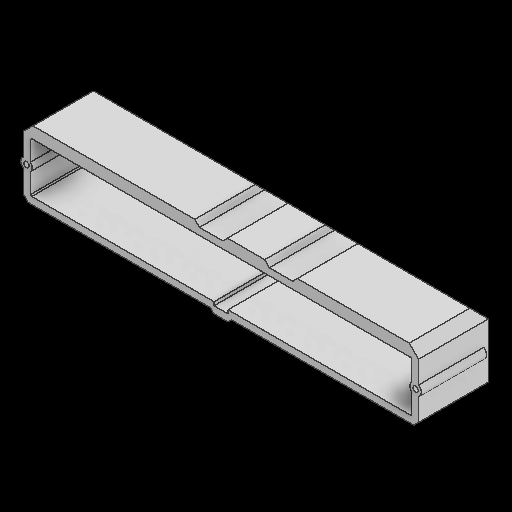
# Autodesk Inventor part: DepthCameraHousing
Saved by Autodesk Inventor 2025.2 (Build 292293000, 293)
## iProperties
Created: 2026-02-04
Part Number: DepthCameraHousing
Material: Generic
Document SubType Name: Modeling
Designer: valer
Density: 1 g/cm^3
Appearance: Default
Author: valer
Autodesk Inventor part; units mm, degrees
ref_plane "YZ Plane" through (0, 0, 0) normal (1, 0, 0) x (0, 1, 0)
ref_plane "XZ Plane" through (0, 0, 0) normal (0, 1, 0) x (-1, 0, 0)
ref_plane "XY Plane" through (0, 0, 0) normal (0, 0, 1) x (1, 0, 0)
sketch "Base" plane through (0, 0, 0) normal (0, 0, 1) x (1, 0, 0)
  line L0 (-81.75, 10.75) -> (81.75, 10.75)
  line L1 (81.75, 10.75) -> (81.75, -10.75)
  line L2 (81.75, -10.75) -> (-81.75, -10.75)
  line L3 (-81.75, -10.75) -> (-81.75, 10.75)
  line L4 (-81.75, 10.75) -> (81.75, -10.75) construction
  line L5 (81.75, 10.75) -> (-81.75, -10.75) construction
  line L6 (-81.75, 10.75) -> (-81.75, 13.75)
  line L7 (-120.4, 0) -> (120.4, 0) construction
  line L8 (0, -19.25) -> (0, 19.25) construction
  line L9 (84.75, 13.75) -> (-84.75, 13.75)
  line L10 (-84.75, 13.75) -> (-84.75, -13.75)
  line L11 (-84.75, -13.75) -> (84.75, -13.75)
  line L12 (84.75, -13.75) -> (84.75, 13.75)
  point P0 (0, 0)
  dimension "d0" = 21.5
  dimension "d1" = 163.5
  dimension "d14" = 3
  constraints: 22 end point, 4 parallel, 2 midpoint, 2 perpendicular, 1 horizontal, 3 other
  measures "d0" distance between parallel lines of L2 L0
  measures "d1" distance of L0.start L0.end
  measures "d14" distance between parallel lines of L0 L9
extrude "BaseFeature" add sketch "Base" along normal blind 27
fillet "InsideFilletsFeature" radius 0.5 4 edges at (-81.75, 10.75, 13.5) (81.75, 10.75, 13.5) (81.75, -10.75, 13.5) (-81.75, -10.75, 13.5)
sketch "Cap" plane through (0, 0, 0) normal (0, 0, -1) x (-1, 0, 0)
  line L0 (84.75, -13.75) -> (-84.75, -13.75) projected
  line L1 (84.75, 13.75) -> (84.75, -13.75) projected
  line L2 (-84.75, 13.75) -> (84.75, 13.75) projected
  line L3 (-84.75, -13.75) -> (-84.75, 13.75) projected
extrude "CapFeature" add sketch "Cap" along normal blind 3
sketch "FrontMount" plane through (0, 0, 0) normal (0, 0, 1) x (1, 0, 0)
  line L0 (-120.4, 0) -> (120.4, 0) construction
  line L1 (0, -19.25) -> (0, 19.25) construction
  circle A0 centre (-83.5, 0) radius 2.5
  circle A1 centre (83.5, 0) radius 2.5
  circle A2 centre (-83.5, 0) radius 1.15
  circle A3 centre (83.5, 0) radius 1.15
  point P0 (0, 0)
  dimension "d11" = 167
  dimension "d12" = 5
  dimension "d13" = 2.3
  constraints: 4 centre point, 2 coincident, 1 equal radius, 1 point on line, 1 symmetric about line, 1 other
  measures "d11" distance of A1.centre A0.centre
  measures "d12" diameter of A0
  measures "d13" diameter of A2
extrude "FrontMountFeature" add sketch "FrontMount" along normal up to surface (27 mm away)
chamfer "SideChamfersFeature" distance 2 angle 45 4 edges at (-84.75, 13.75, 12) (84.75, 13.75, 12) (-84.75, -13.75, 12) (84.75, -13.75, 12)
chamfer "BackChamferFeature" distance 2 angle 45 8 edges at (0, 13.75, -3) (-83.75, 12.75, -3) (-84.75, 0, -3) (-83.75, -12.75, -3) (0, -13.75, -3) (83.75, 12.75, -3) (84.75, 0, -3) (83.75, -12.75, -3)
sketch "FrontMountHoles" plane through (0, 0, 27) normal (0, 0, 1) x (1, 0, 0)
  arc A0 (-84.75, 2.1651) -> (-84.75, -2.1651) centre (-83.5, 0) ccw projected
  arc A1 (84.75, -2.1651) -> (84.75, 2.1651) centre (83.5, 0) ccw projected
  arc A2 (-81.75, -1.7854) -> (-81.75, 1.7854) centre (-83.5, 0) ccw projected
  circle A3 centre (-83.5, 0) radius 1.175
  circle A4 centre (83.5, 0) radius 1.175
  point P0 (0, 0)
  dimension "d20" = 2.35
  dimension "d21" = 2.35
  constraints: 2 centre point, 2 coincident
  measures "d20" diameter of A3
  measures "d21" diameter of A4
extrude "FrontMountHolesFeature" cut sketch "FrontMountHoles" against normal blind 15
sketch "BackEndExtrusion" plane through (0, 0, 0) normal (0, 0, -1) x (-1, 0, 0)
  line L0 (84.75, -2.1651) -> (84.75, 2.1651) projected
  arc A0 (84.75, -2.1651) -> (84.75, 2.1651) centre (83.5, 0) ccw projected
  line L1 (-84.75, 2.1651) -> (-84.75, -2.1651) projected
  arc A1 (-84.75, 2.1651) -> (-84.75, -2.1651) centre (-83.5, 0) ccw projected
  point P0 (0, 0)
extrude "BackEndExtrusionFeature" add sketch "BackEndExtrusion" along normal up to surface (1 mm away)
sketch "CableIndent" plane through (0, 0, 27) normal (0, 0, 1) x (1, 0, 0)
  line L0 (0, -19.25) -> (0, 19.25) construction
  line L1 (81.25, -10.75) -> (-81.25, -10.75) projected
  line L2 (-3, -10.75) -> (-3, -12.25)
  line L3 (-3, -12.25) -> (3, -12.25)
  line L4 (3, -12.25) -> (3, -10.75)
  point P0 (0, 0)
  point P1 (0, -12.25)
  dimension "d29" = 6
  dimension "d30" = 1.5
  constraints: 6 end point, 3 point on line, 2 perpendicular, 1 midpoint, 1 vertical
  measures "d29" distance of L2.end L3.end
  measures "d30" distance of L3.end L4.end
extrude "CableIndentFeature" cut sketch "CableIndent" against normal up to surface (27 mm away)
sketch "Sketch7" plane through (0, 0, 27) normal (0, 0, 1) x (1, 0, 0)
  line L0 (82.75, 13.75) -> (-82.75, 13.75) projected
  line L1 (-82.75, 13.75) -> (-80.75, 15.75)
  line L2 (-80.75, 15.75) -> (-11.25, 15.75)
  line L3 (-11.25, 15.75) -> (-9.25, 13.75)
  line L4 (82.75, 13.75) -> (80.75, 15.75)
  line L5 (80.75, 15.75) -> (32.75, 15.75)
  line L6 (32.75, 15.75) -> (30.75, 13.75)
  line L7 (30.75, 13.75) -> (20.75, 13.75)
  line L8 (20.75, 13.75) -> (18.75, 15.75)
  line L9 (18.75, 15.75) -> (2.75, 15.75)
  line L10 (2.75, 15.75) -> (0.75, 13.75)
  line L11 (82.75, 13.75) -> (84.75, 11.75) projected
  line L12 (-84.75, 11.75) -> (-82.75, 13.75) projected
  point P0 (0, 0)
  dimension "d33" = 0
  dimension "d34" = 2
  dimension "d35" = 45
  dimension "d36" = 45
  dimension "d37" = 45
  dimension "d38" = 45
  dimension "d39" = 45
  dimension "d40" = 52
  dimension "d41" = 10
  dimension "d42" = 20
  dimension "d44" = 10
  constraints: 20 end point, 4 parallel, 4 point on line, 3 collinear, 2 perpendicular, 1 horizontal
  measures "d33" distance between parallel lines of L0 L7
  measures "d34" distance between parallel lines of L5 L0
  measures "d35" angle of L0 L4
  measures "d36" angle of L0 L6
  measures "d37" angle of L0 L8
  measures "d38" angle of L0 L10
  measures "d39" angle of L0 L3
  measures "d40" distance of L0.start L6.end
  measures "d41" distance of L6.end L7.end
  measures "d42" distance of L10.end L7.end
  measures "d44" distance of L10.end L3.end
extrude "Extrusion7" add sketch "Sketch7" against normal up to surface (28 mm away)
delete faces "Delete1" heal yes whole lump no faces at (48.75, 14.4167, -1) (8.0833, 14.4167, -1) (-34.4167, 14.4167, -1)
delete faces "Delete2" heal yes whole lump no faces at (-83.4167, 12.1405, -1.6667) (83.1405, 12.4167, -1.6667)
delete faces "Delete3" heal yes whole lump no faces at (-83.4167, 0.9978, -2.3333) (-83.4167, -12.1405, -1.6667) (-27.3072, -13.0833, -1.6667) (83.4167, 0.9978, -2.3333) (83.1405, -12.4167, -1.6667)
sketch "Sketch8" plane through (0, 0, 27) normal (0, 0, 1) x (1, 0, 0)
  line L0 (-82.75, -13.75) -> (82.75, -13.75) projected
  line L1 (-4.5, -13.75) -> (-3, -15.25)
  line L2 (-3, -15.25) -> (3, -15.25)
  line L3 (3, -15.25) -> (4.5, -13.75)
  line L4 (0, -22.0092) -> (0, 22.0432) construction
  line L5 (3, -12.25) -> (-3, -12.25) projected
  line L6 (-3, -12.25) -> (-3, -15.25) construction
  point P0 (0, 0)
  point P1 (0, -15.25)
  dimension "d47" = 1.5
  dimension "d48" = 135
  constraints: 8 end point, 3 point on line, 2 perpendicular, 1 midpoint, 1 parallel
  measures "d47" distance between parallel lines of L2 L0
  measures "d48" angle of L2 L1
extrude "Extrusion8" add sketch "Sketch8" against normal up to surface (30 mm away)
body "Solid1"
